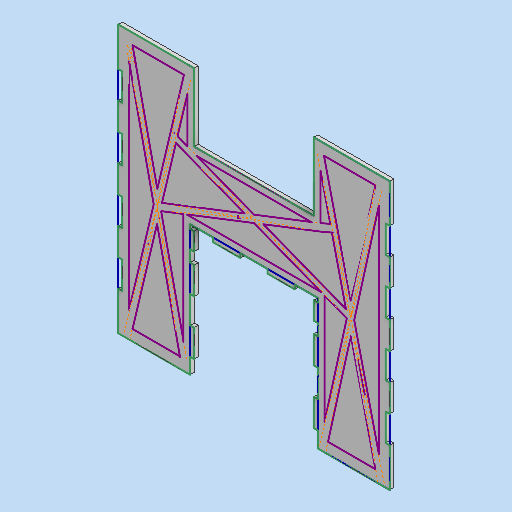
# Autodesk Inventor part: back plate
Saved by Autodesk Inventor 2026 (Build 300175000, 175)
## iProperties
Created: 2026-02-11
Part Number: back plate
Material: Generic
Document SubType Name: Modeling
Designer: mones
Density: 1 g/cm^3
Appearance: Default
Author: mones
Autodesk Inventor part; units mm, degrees
ref_plane "YZ Plane" through (0, 0, 0) normal (1, 0, 0) x (0, 1, 0)
ref_plane "XZ Plane" through (0, 0, 0) normal (0, 1, 0) x (-1, 0, 0)
ref_plane "XY Plane" through (0, 0, 0) normal (0, 0, 1) x (1, 0, 0)
sketch "Sketch1" plane through (0, 0, 0) normal (0, 0, 1) x (1, 0, 0)
  line L0 (-100, 98.5) -> (100, -98.5) construction
  line L1 (100, 98.5) -> (-100, -98.5) construction
  line L2 (-100, 98.5) -> (-100, 70)
  line L3 (-100, 50) -> (-100, 30)
  line L4 (-100, 10) -> (-100, -10)
  line L5 (-100, -30) -> (-100, -50)
  line L6 (-100, -70) -> (-100, -98.5)
  line L7 (-100, 98.5) -> (-100, 95.5)
  line L8 (-100, 98.5) -> (-100, 95.5)
  line L9 (-100, 98.5) -> (-97, 98.5)
  line L10 (-100, -70) -> (-97, -70)
  line L11 (-100, -50) -> (-97, -50)
  line L12 (-100, -30) -> (-97, -30)
  line L13 (-100, -10) -> (-97, -10)
  line L14 (-100, 10) -> (-97, 10)
  line L15 (-100, 30) -> (-97, 30)
  line L16 (-100, 50) -> (-97, 50)
  line L17 (-100, 70) -> (-97, 70)
  line L18 (-100, -98.5) -> (-100, -70)
  line L19 (-100, -50) -> (-100, -30)
  line L20 (-100, -10) -> (-100, 10)
  line L21 (-100, 30) -> (-100, 50)
  line L22 (-100, 70) -> (-100, 98.5)
  line L23 (100, 98.5) -> (97, 98.5)
  line L24 (100, -98.5) -> (100, -70)
  line L25 (100, -50) -> (100, -30)
  line L26 (100, -10) -> (100, 10)
  line L27 (100, 30) -> (100, 50)
  line L28 (100, 70) -> (97, 70)
  line L29 (100, 50) -> (97, 50)
  line L30 (100, 30) -> (97, 30)
  line L31 (100, 10) -> (97, 10)
  line L32 (100, -10) -> (97, -10)
  line L33 (100, -30) -> (97, -30)
  line L34 (100, -50) -> (97, -50)
  line L35 (100, -70) -> (97, -70)
  line L36 (100, -70) -> (100, -98.5)
  line L37 (100, -30) -> (100, -50)
  line L38 (100, 10) -> (100, -10)
  line L39 (100, 98.5) -> (100, 70)
  line L40 (100, 50) -> (100, 30)
  line L41 (-97, -98.5) -> (-47, -98.5)
  line L42 (-47, -98.5) -> (-100, -98.5)
  line L43 (-100, 98.5) -> (-47, 98.5)
  line L44 (100, -98.5) -> (47, -98.5)
  line L45 (47, -98.5) -> (47, -87)
  line L46 (47, -87) -> (47, -98.5)
  line L47 (100, -98.5) -> (47, -98.5)
  line L48 (47, 98.5) -> (97, 98.5)
  line L49 (47, 98.5) -> (100, 98.5)
  line L50 (-97, 98.5) -> (-47, 98.5)
  line L51 (-97, 70) -> (-97, 50)
  line L52 (-97, 30) -> (-97, 10)
  line L53 (-97, -10) -> (-97, -30)
  line L54 (-97, -50) -> (-97, -70)
  line L55 (97, -50) -> (97, -70)
  line L56 (97, -10) -> (97, -30)
  line L57 (97, 30) -> (97, 10)
  line L58 (97, 70) -> (97, 50)
  line L59 (-44, -68.5) -> (-44, -67)
  line L60 (-44, 71.5) -> (-44, 51.5)
  line L61 (-44, 48.5) -> (44, 48.5)
  line L62 (44, 51.5) -> (44, 71.5)
  line L63 (44, 71.5) -> (44, 98.5)
  line L64 (-44, 71.5) -> (-44, 98.5)
  line L65 (-44, 51.5) -> (-44, 48.5)
  line L66 (44, 51.5) -> (44, 48.5)
  line L67 (47, -98.5) -> (47, -87)
  line L68 (47, -87) -> (44, -87)
  line L69 (44, -87) -> (44, -67)
  line L70 (44, -67) -> (47, -67)
  line L71 (44, -47) -> (47, -47)
  line L72 (44, -27) -> (47, -27)
  line L73 (44, -18.5) -> (47, -18.5)
  line L74 (44, -87) -> (44, -67)
  line L75 (47, -67) -> (47, -47)
  line L76 (47, -27) -> (47, -18.5)
  line L77 (-44, -87) -> (-44, -68.5)
  line L78 (47, 98.5) -> (44, 98.5)
  line L79 (-44, 98.5) -> (-47, 98.5)
  line L80 (-47, -87) -> (-47, -98.5)
  line L81 (-47, -98.5) -> (-47, -87)
  line L82 (-47, -98.5) -> (-47, -87)
  line L83 (-47, -87) -> (-44, -87)
  line L84 (-44, -87) -> (-44, -67)
  line L85 (-44, -67) -> (-47, -67)
  line L86 (-44, -47) -> (-47, -47)
  line L87 (-44, -27) -> (-47, -27)
  line L88 (-44, -18.5) -> (-47, -18.5)
  line L89 (-44, -87) -> (-44, -67)
  line L90 (-47, -67) -> (-47, -47)
  line L91 (-47, -27) -> (-47, -18.5)
  line L92 (-47, -98.5) -> (-47, -87)
  line L93 (47, -67) -> (47, -47)
  line L94 (47, -47) -> (47, -47.4373)
  line L95 (44, -47) -> (44, -27)
  line L96 (44, -18.5) -> (44, -6.5)
  line L97 (-44, -18.5) -> (-44, -6.5)
  line L98 (-44, -47) -> (-44, -27)
  line L99 (47, -27) -> (47, -18.5)
  line L100 (-47, -27) -> (-47, -18.5)
  line L101 (-47, -98.5) -> (-47, -87)
  line L102 (-47, -67) -> (-47, -47)
  line L103 (-47, -5.5) -> (-47, -2.5)
  line L104 (-44, -6.5) -> (-44, -5.5)
  line L105 (-44, -5.5) -> (-47, -5.5)
  line L106 (44, -6.5) -> (44, -5.5)
  line L107 (44, -5.5) -> (47, -5.5)
  line L108 (47, -5.5) -> (47, -2.5)
  line L109 (-47, -2.5) -> (-30, -2.5)
  line L110 (-10, -2.5) -> (10, -2.5)
  line L111 (30, -2.5) -> (47, -2.5)
  line L112 (-30, -2.5) -> (-30, -5.5)
  line L113 (-10, -2.5) -> (-10, -5.5)
  line L114 (10, -2.5) -> (10, -5.5)
  line L115 (30, -2.5) -> (30, -5.5)
  line L116 (30, -5.5) -> (10, -5.5)
  line L117 (-10, -5.5) -> (-30, -5.5)
  line L118 (47, -2.5) -> (30, -2.5)
  line L119 (10, -2.5) -> (-10, -2.5)
  line L120 (-30, -2.5) -> (-47, -2.5)
  constraints: 242 end point, 84 perpendicular, 38 parallel, 10 vertical, 7 collinear, 7 horizontal, 4 point on line
extrude "Extrusion1" add sketch "Sketch1" along normal blind 3
sketch "Sketch3" plane through (0, 0, 3) normal (0, 0, 1) x (1, 0, 0)
  line L0 (-100, -70) -> (-100, -98.5) projected
  line L1 (-100, -98.5) -> (-47, -98.5) projected
  line L2 (-47, -98.5) -> (-47, -87) projected
  line L3 (-47, -87) -> (-44, -87) projected
  line L4 (-44, -87) -> (-44, -67) projected
  line L5 (-44, -67) -> (-47, -67) projected
  line L6 (-47, -67) -> (-47, -47) projected
  line L7 (-47, -47) -> (-44, -47) projected
  line L8 (-44, -47) -> (-44, -27) projected
  line L9 (-44, -27) -> (-47, -27) projected
  line L10 (-47, -27) -> (-47, -18.5) projected
  line L11 (-47, -18.5) -> (-44, -18.5) projected
  line L12 (-44, -18.5) -> (-44, -5.5) projected
  line L13 (-44, -5.5) -> (-47, -5.5) projected
  line L14 (-47, -5.5) -> (-47, -2.5) projected
  line L15 (-47, -2.5) -> (-30, -2.5) projected
  line L16 (-30, -2.5) -> (-30, -5.5) projected
  line L17 (-30, -5.5) -> (-10, -5.5) projected
  line L18 (-10, -5.5) -> (-10, -2.5) projected
  line L19 (-10, -2.5) -> (10, -2.5) projected
  line L20 (10, -2.5) -> (10, -5.5) projected
  line L21 (10, -5.5) -> (30, -5.5) projected
  line L22 (30, -5.5) -> (30, -2.5) projected
  line L23 (30, -2.5) -> (47, -2.5) projected
  line L24 (47, -2.5) -> (47, -5.5) projected
  line L25 (47, -5.5) -> (44, -5.5) projected
  line L26 (44, -5.5) -> (44, -18.5) projected
  line L27 (44, -18.5) -> (47, -18.5) projected
  line L28 (47, -18.5) -> (47, -27) projected
  line L29 (47, -27) -> (44, -27) projected
  line L30 (44, -27) -> (44, -47) projected
  line L31 (44, -47) -> (47, -47) projected
  line L32 (47, -47) -> (47, -67) projected
  line L33 (47, -67) -> (44, -67) projected
  line L34 (44, -67) -> (44, -87) projected
  line L35 (44, -87) -> (47, -87) projected
  line L36 (47, -87) -> (47, -98.5) projected
  line L37 (47, -98.5) -> (100, -98.5) projected
  line L38 (100, -98.5) -> (100, -70) projected
  line L39 (100, -70) -> (97, -70) projected
  line L40 (97, -70) -> (97, -50) projected
  line L41 (97, -50) -> (100, -50) projected
  line L42 (100, -50) -> (100, -30) projected
  line L43 (100, -30) -> (97, -30) projected
  line L44 (97, -30) -> (97, -10) projected
  line L45 (97, -10) -> (100, -10) projected
  line L46 (100, -10) -> (100, 10) projected
  line L47 (100, 10) -> (97, 10) projected
  line L48 (97, 10) -> (97, 30) projected
  line L49 (97, 30) -> (100, 30) projected
  line L50 (100, 30) -> (100, 50) projected
  line L51 (100, 50) -> (97, 50) projected
  line L52 (97, 50) -> (97, 70) projected
  line L53 (97, 70) -> (100, 70) projected
  line L54 (100, 70) -> (100, 98.5) projected
  line L55 (100, 98.5) -> (44, 98.5) projected
  line L56 (44, 98.5) -> (44, 48.5) projected
  line L57 (44, 48.5) -> (-44, 48.5) projected
  line L58 (-44, 48.5) -> (-44, 98.5) projected
  line L59 (-44, 98.5) -> (-100, 98.5) projected
  line L60 (-100, 98.5) -> (-100, 70) projected
  line L61 (-100, 70) -> (-97, 70) projected
  line L62 (-97, 70) -> (-97, 50) projected
  line L63 (-97, 50) -> (-100, 50) projected
  line L64 (-100, 50) -> (-100, 30) projected
  line L65 (-100, 30) -> (-97, 30) projected
  line L66 (-97, 30) -> (-97, 10) projected
  line L67 (-97, 10) -> (-100, 10) projected
  line L68 (-100, 10) -> (-100, -10) projected
  line L69 (-100, -10) -> (-97, -10) projected
  line L70 (-97, -10) -> (-97, -30) projected
  line L71 (-97, -30) -> (-100, -30) projected
  line L72 (-100, -30) -> (-100, -50) projected
  line L73 (-100, -50) -> (-97, -50) projected
  line L74 (-97, -50) -> (-97, -70) projected
  line L75 (-97, -70) -> (-100, -70) projected
  line L76 (100, 98.5) -> (100, -98.5)
  line L77 (100, -98.5) -> (52, -98.5)
  line L78 (-100, -98.5) -> (-100, 98.5)
  line L79 (92, -79.6839) -> (92, 78.9145)
  line L80 (44, 70) -> (44, 48.5)
  line L81 (44, 48.5) -> (-44, 48.5)
  line L82 (-44, 90.5) -> (-44, 98.5)
  line L83 (-42.102, 43.5) -> (42.727, 43.5)
  line L84 (-47, -2.5) -> (47, -2.5)
  line L85 (47, -2.5) -> (47, -98.5)
  line L86 (89.4543, 90.5) -> (51.5538, 90.5)
  line L87 (-51.5537, 90.5) -> (-89.4397, 90.5)
  line L88 (-49, 98.5) -> (-44, 98.5)
  line L89 (44, 98.5) -> (100, 98.5)
  line L90 (-49, 79.6839) -> (-49, 46.1824)
  line L91 (-52, 1.5427) -> (-52, -80.2167)
  line L92 (-89.6243, -90.5) -> (-54.5446, -90.5)
  line L93 (54.5603, -90.5) -> (89.4304, -90.5)
  line L94 (-47, -87) -> (-47, -2.5)
  line L95 (48.1131, -96.5027) -> (94.4411, 89.9605) construction
  line L96 (89.5589, 91.0395) -> (52.9953, -97.5816) construction
  line L97 (91.1219, -97.62) -> (51.4323, 91.0778) construction
  line L98 (46.5677, 89.9222) -> (95.9865, -96.4643) construction
  line L99 (-48.0939, 45.83) -> (70.371, -5.6011) construction
  line L100 (72.1832, -0.9411) -> (-49.9061, 41.17) construction
  line L101 (-72.1832, -0.9411) -> (49.9061, 41.17) construction
  line L102 (49, 46.2234) -> (56.206, 49.3518)
  line L103 (58.1956, 44.7689) -> (50.0836, 41.2471)
  line L104 (-57.4526, 44.1045) -> (-49.9061, 41.17)
  line L105 (-95.9865, -96.4643) -> (-46.5677, 89.9222) construction
  line L106 (-51.4322, 91.0779) -> (-91.1219, -97.62) construction
  line L107 (-92.9953, 83.4184) -> (-49.5589, -89.9605) construction
  line L108 (-54.4411, -91.0395) -> (-88.113, 84.4973) construction
  line L109 (-52, -78.9146) -> (-68.3735, -4.8244)
  line L110 (-52, 1.5427) -> (-68.3735, -4.8244)
  line L111 (-71.3652, -14.458) -> (-89.4304, -90.5)
  line L112 (-71.1889, 7.9158) -> (-88.113, 84.4973)
  line L113 (-71.1889, 7.9158) -> (-51.5695, 90.5)
  line L114 (-92, -79.6839) -> (-73.8419, -3.2509)
  line L115 (-92, 78.9146) -> (-73.8419, -3.2509)
  line L116 (-71.3652, -14.458) -> (-54.4411, -91.0395)
  line L117 (-69.7951, -9.977) -> (-69.7901, -10)
  line L118 (-77.699, -30.3026) -> (-77.6271, -30)
  line L119 (-89.4397, 90.5) -> (-86.6673, 77.9551)
  line L120 (-91.5495, 76.8762) -> (-89.5589, 91.0395) construction
  line L121 (-94.4411, 89.9605) -> (-86.6673, 77.9551) construction
  line L122 (-92, 78.9146) -> (-92, -79.6839)
  line L123 (-91.5495, 76.8762) -> (-92, 78.9146)
  line L124 (-49, 90.5) -> (-48.9998, 90.5)
  line L125 (-49, 46.1824) -> (-56.2858, 49.0155)
  line L126 (-58.6381, 49.9303) -> (-58.695, 49.9524)
  line L127 (-49, 79.6839) -> (-56.2858, 49.0155)
  line L128 (-57.4526, 44.1045) -> (-67.7439, 0.7852)
  line L129 (-67.7439, 0.7852) -> (-6.898, 24.4458)
  line L130 (0, 27.1282) -> (42.102, 43.5)
  line L131 (-42.102, 43.5) -> (0, 27.1282)
  line L132 (-6.898, 24.4458) -> (-49.9061, 41.17)
  line L133 (48.0939, 45.83) -> (42.727, 43.5) construction
  line L134 (0, 24.9502) -> (-70.371, -5.6011) construction
  line L135 (49.9061, 41.17) -> (6.898, 24.4458)
  line L136 (0, 21.7634) -> (-49.5381, 2.5)
  line L137 (49, 46.2234) -> (49, 79.6839)
  line L138 (56.206, 49.3518) -> (49, 79.6839)
  line L139 (49.5381, 2.5) -> (-49.5381, 2.5)
  line L140 (49.5381, 2.5) -> (0, 21.7634)
  line L141 (67.7439, 0.7852) -> (57.379, 44.4143)
  line L142 (52, -78.9145) -> (68.3735, -4.8244)
  line L143 (6.898, 24.4458) -> (67.7439, 0.7852)
  line L144 (71.189, 7.9158) -> (89.4397, 90.5)
  line L145 (51.5696, 90.5) -> (71.189, 7.9158)
  line L146 (73.8419, -3.2509) -> (92, -79.6839)
  line L147 (68.3735, -4.8244) -> (52, 1.5427)
  line L148 (92, 78.9145) -> (73.8419, -3.2509)
  line L149 (76.9144, -27) -> (81.6657, -47)
  line L150 (71.3652, -14.458) -> (54.5603, -90.5)
  line L151 (89.4304, -90.5) -> (71.3652, -14.458)
  line L152 (52, -78.9145) -> (52, 1.5427)
  point P0 (-11.1386, 20.1145)
  constraints: 156 end point, 55 parallel, 23 point on line, 8 perpendicular, 3 horizontal, 1 midpoint
body "Solid1"
